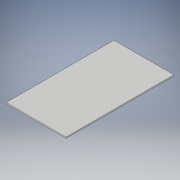
# Autodesk Inventor part: caixa interruptors_tapa
Saved by Autodesk Inventor 2019 (Build 230136000, 136)
## iProperties
Created: 2018-08-12
Part Number: caixa interruptors_tapa
Material: Genérico
Document SubType Name: Modeling
Designer: Albert Garangou Culebras
Density: 1 g/cm^3
Appearance: Valor por defecto
Author: Albert Garangou Culebras
Autodesk Inventor part; units mm, degrees
ref_plane "YZ Plane" through (0, 0, 0) normal (1, 0, 0) x (0, 1, 0)
ref_plane "XZ Plane" through (0, 0, 0) normal (0, 1, 0) x (-1, 0, 0)
ref_plane "XY Plane" through (0, 0, 0) normal (0, 0, 1) x (1, 0, 0)
sketch "Boceto1" plane through (0, 0, 0) normal (0, 1, 0) x (-1, 0, 0)
  line L0 (0, 0) -> (0, -180)
  line L1 (0, -180) -> (100, -180)
  line L2 (100, -180) -> (100, 0)
  line L3 (100, 0) -> (0, 0)
  dimension "d0" = 180
  dimension "d1" = 100
  dimension "d2" = 90
  constraints: 8 end point, 2 perpendicular, 2 vertical
  measures "d0" distance of L0.start L0.end
  measures "d1" distance of L0.end L1.end
  measures "d2" angle of L1 L0
extrude "Extrusión14" add sketch "Boceto1" along normal blind 2
sketch "Boceto15" plane through (0, 0, 0) normal (0, -1, 0) x (1, 0, 0)
  line L0 (0, 0) -> (0, -2.5)
  line L1 (0, 0) -> (0, -180) projected
  line L2 (0, -2.5) -> (-2.5, -2.5)
  line L3 (-100, 0) -> (-97.5, 0)
  line L4 (-100, 0) -> (0, 0) projected
  line L5 (-97.5, 0) -> (-95, 0)
  line L6 (-97.5, 0) -> (-97.5, -2.5)
  line L7 (-100, -180) -> (-100, 0) projected
  line L8 (-100, -180) -> (-97.5, -180)
  line L9 (0, -180) -> (-100, -180) projected
  line L10 (-97.5, -180) -> (-97.5, -177.5)
  line L11 (0, -180) -> (0, -177.5)
  line L12 (0, -177.5) -> (-2.5, -177.5)
  line L13 (-2.5, -177.5) -> (-97.5, -177.5)
  line L14 (-97.5, -177.5) -> (-97.5, -2.5)
  line L15 (-97.5, -2.5) -> (-2.5, -2.5)
  line L16 (-2.5, -2.5) -> (-2.5, -177.5)
  dimension "d56" = 2.5
  dimension "d57" = 2.5
  dimension "d58" = 2.5
  dimension "d59" = 2.5
  dimension "d60" = 2.5
  dimension "d61" = 2.5
  dimension "d62" = 2.5
  dimension "d63" = 2.5
  dimension "d64" = 2.5
  constraints: 26 end point, 5 point on line, 4 perpendicular, 2 parallel, 1 horizontal, 1 vertical
  measures "d56" distance of L0.start L0.end
  measures "d57" distance of L0.end L2.end
  measures "d58" distance of L3.start L3.end
  measures "d59" distance of L3.end L5.end
  measures "d60" distance of L3.end L6.end
  measures "d61" distance of L7.start L8.end
  measures "d62" distance of L8.end L10.end
  measures "d63" distance of L1.end L11.end
  measures "d64" distance of L11.end L12.end
extrude "Extrusión15" add sketch "Boceto15" along normal blind 2 contours L16 L13 L14 L15
